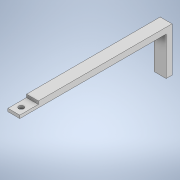
# Autodesk Inventor part: brace1
Saved by Autodesk Inventor 2020.2 (Build 242310000, 310)
## iProperties
Created: 2020-02-12
Part Number: brace1
Material: Generic
Document SubType Name: Modeling
Designer: ColinP
Density: 1 g/cm^3
Appearance: Default
Author: ColinP
Autodesk Inventor part; units mm, degrees
ref_plane "YZ Plane" through (0, 0, 0) normal (1, 0, 0) x (0, 1, 0)
ref_plane "XZ Plane" through (0, 0, 0) normal (0, 1, 0) x (-1, 0, 0)
ref_plane "XY Plane" through (0, 0, 0) normal (0, 0, 1) x (1, 0, 0)
sketch "Sketch1" plane through (0, 0, 0) normal (0, 1, 0) x (-1, 0, 0)
  line L0 (0, 0) -> (8, 0)
  line L1 (8, 0) -> (8, 98.806)
  line L2 (8, 98.806) -> (0, 98.806)
  line L3 (0, 98.806) -> (0, 0)
  line L4 (4, 0) -> (4, 98.806)
  line L5 (4, 98.806) -> (4, 93.806)
  circle A0 centre (4, 93.806) radius 1.7
  dimension "d0" = 8
  dimension "d1" = 98.806
  dimension "d2" = 90
  dimension "d3" = 8
  dimension "d4" = 98.806
  dimension "d5" = 5
  dimension "d6" = 3.4
  constraints: 12 end point, 2 midpoint, 2 perpendicular, 1 centre point, 1 coincident, 1 horizontal, 1 point on line
  measures "d0" distance of L0.start L0.end
  measures "d1" distance of L0.end L1.end
  measures "d2" angle of L1 L0
  measures "d3" distance of L1.end L2.end
  measures "d4" distance of L4.start L4.end
  measures "d5" distance of L4.end L5.end
  measures "d6" diameter of A0
extrude "Extrusion1" add sketch "Sketch1" along normal blind 4 contours L3 L2 L4 A0 L0 | L4 A0 L2 L1 L0
sketch "Sketch2" plane through (-8, 0, 98.806) normal (0, 0, 1) x (1, 0, 0)
  line L0 (8, 4) -> (0, 4) projected
  line L1 (0, 4) -> (8, 4)
  line L2 (8, 4) -> (8, 2)
  line L3 (8, 2) -> (0, 2)
  line L4 (0, 2) -> (0, 4)
  point P0 (8, 0)
  dimension "d9" = 8
  dimension "d10" = 2
  constraints: 8 end point, 2 parallel, 1 horizontal, 1 perpendicular
  measures "d9" distance of L2.end L3.end
  measures "d10" distance of L1.end L2.end
extrude "Extrusion2" cut sketch "Sketch2" against normal blind 12.54
sketch "Sketch3" plane through (0, 4, 0) normal (0, 1, 0) x (1, 0, 0)
  line L0 (0, 0) -> (-8, 0) projected
  line L1 (0, 0) -> (-8, 0)
  line L2 (-8, 0) -> (-8, 4)
  line L3 (-8, 4) -> (0, 4)
  line L4 (0, 4) -> (0, 0)
  dimension "d13" = 8
  dimension "d14" = 4
  constraints: 8 end point, 2 parallel, 1 horizontal, 1 perpendicular
  measures "d13" distance of L2.end L3.end
  measures "d14" distance of L1.end L2.end
extrude "Extrusion3" add sketch "Sketch3" against normal blind 30
body "Solid1"
